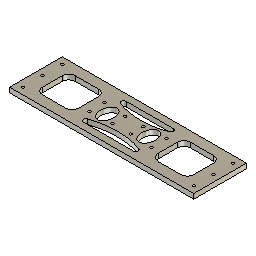
Mark3_new_z_vertical_bracket (Autodesk Fusion 360 design; units mm, degrees)
Autodesk Fusion 360 part; units mm, degrees
note: some values were not read from the file. Set by a fixed rule: which face or edge a step refers to.
sketch "Sketch1" plane through (0, 0, 0) normal (0, 0, 1) x (1, 0, 0)
  line L0 (17.5, -12.12) -> (-17.5, -12.12)
  line L1 (-17.5, -12.12) -> (-17.5, 12.12)
  line L2 (-17.5, 12.12) -> (17.5, 12.12)
  line L3 (17.5, 12.12) -> (17.5, -12.12)
  line L4 (17.5, -12.12) -> (-17.5, 12.12) construction
  line L5 (-17.5, -12.12) -> (17.5, 12.12) construction
  line L6 (114.3, -31.75) -> (-114.3, -31.75)
  line L7 (-114.3, -31.75) -> (-114.3, 31.75)
  line L8 (-114.3, 31.75) -> (114.3, 31.75)
  line L9 (114.3, 31.75) -> (114.3, -31.75)
  ellipse E0 centre (-38.75, 1.2425) end of major axis (-38.75, -20.9825) minor radius 13.97
  line L10 (-38.75, 23.4675) -> (-38.75, -20.9825)
  line L11 (-52.72, 1.2425) -> (-24.78, 1.2425)
  ellipse E1 centre (38.75, 1.2425) end of major axis (38.75, -20.9825) minor radius 13.97
  line L12 (38.75, 23.4675) -> (38.75, -20.9825)
  line L13 (24.78, 1.2425) -> (52.72, 1.2425)
  line L14 (635, -50.8) -> (279.4, -50.8)
  line L15 (279.4, -50.8) -> (279.4, 50.8)
  line L16 (279.4, 50.8) -> (635, 50.8)
  line L17 (635, 50.8) -> (635, -50.8)
  line L18 (635, -50.8) -> (279.4, 50.8) construction
  line L19 (279.4, -50.8) -> (635, 50.8) construction
  line L20 (381, -19.05) -> (381, 19.05)
  line L21 (533.4, 16.51) -> (533.4, -19.05)
  line L22 (533.4, -31.75) -> (381, 31.75) construction
  line L23 (381, -31.75) -> (533.4, 31.75) construction
  line L24 (311.15, 19.05) -> (311.15, -19.05)
  line L25 (603.25, -19.05) -> (603.25, 19.05)
  line L26 (603.25, 31.75) -> (311.15, -31.75) construction
  line L27 (311.15, 31.75) -> (603.25, -31.75) construction
  line L28 (590.55, 31.75) -> (548.64, 31.75)
  line L29 (368.3, 31.75) -> (323.85, 31.75)
  line L30 (323.85, -31.75) -> (368.3, -31.75)
  line L31 (546.1, -31.75) -> (590.55, -31.75)
  arc A0 (548.64, 31.75) -> (533.4, 16.51) centre (548.64, 16.51) ccw
  arc A1 (603.25, 19.05) -> (590.55, 31.75) centre (590.55, 19.05) ccw
  arc A2 (590.55, -31.75) -> (603.25, -19.05) centre (590.55, -19.05) ccw
  arc A3 (533.4, -19.05) -> (546.1, -31.75) centre (546.1, -19.05) ccw
  arc A4 (381, 19.05) -> (368.3, 31.75) centre (368.3, 19.05) ccw
  arc A5 (323.85, 31.75) -> (311.15, 19.05) centre (323.85, 19.05) ccw
  arc A6 (311.15, -19.05) -> (323.85, -31.75) centre (323.85, -19.05) ccw
  arc A7 (368.3, -31.75) -> (381, -19.05) centre (368.3, -19.05) ccw
  line L32 (457.2, -38.1) -> (528.32, -38.1)
  line L33 (457.2, -38.1) -> (393.7, -38.1)
  arc A8 (528.32, -38.1) -> (393.7, -38.1) centre (461.01, -156.5222) ccw
  line L34 (457.2, 38.1) -> (528.32, 38.1)
  line L35 (457.2, 38.1) -> (386.08, 38.1)
  arc A9 (386.08, 38.1) -> (528.32, 38.1) centre (457.2, 171.45) ccw
  ellipse E2 centre (418.45, 1.2425) end of major axis (418.45, -17.8075) minor radius 12.7
  line L36 (418.45, 20.2925) -> (418.45, -17.8075)
  line L37 (405.75, 1.2425) -> (431.15, 1.2425)
  ellipse E3 centre (495.95, -1.2425) end of major axis (495.95, -20.2925) minor radius 12.7
  line L38 (495.95, 17.8075) -> (495.95, -20.2925)
  line L39 (483.25, -1.2425) -> (508.65, -1.2425)
  point P0 (-60, 14.605)
  point P1 (-60, -14.605)
  point P2 (17.5, -12.12)
  point P3 (17.5, 12.12)
  point P4 (-17.5, 12.12)
  point P5 (-17.5, -12.12)
  point P6 (60, 14.605)
  point P7 (60, -14.605)
  point P8 (-114.3, 31.75)
  point P9 (114.3, 31.75)
  point P10 (114.3, -31.75)
  point P11 (-114.3, -31.75)
  point P12 (-38.75, 1.2425)
  point P13 (38.75, 1.2425)
  point P14 (457.2, 0)
  point P15 (517.2, 14.605)
  point P16 (517.2, -14.605)
  point P17 (439.7, -12.12)
  point P18 (397.2, -14.605)
  point P19 (397.2, 14.605)
  point P20 (474.7, -12.12)
  point P21 (474.7, 12.12)
  point P22 (457.2, 0)
  point P23 (457.2, 0)
  point P24 (439.7, 12.12)
  point P25 (457.2, 0)
  point P26 (418.45, 1.2425)
  point P27 (457.2, 0)
  point P28 (292.1, 38.1)
  point P29 (292.1, -38.1)
  point P30 (622.3, -38.1)
  point P31 (622.3, 38.1)
  point P32 (292.1, 0)
  point P33 (622.3, 0)
  point P34 (397.2, 14.605)
  point P35 (397.2, -14.605)
  point P36 (517.2, -14.605)
  point P37 (517.2, 14.605)
  point P38 (457.2, 0)
  point P39 (457.2, 0)
  point P40 (457.2, 0)
  point P41 (418.45, 1.2425)
  point P42 (495.95, -1.2425)
  point P43 (457.2, -50.8)
  point P44 (457.2, 50.8)
  dimension "d1" = 24.24
  dimension "d2" = 35
  dimension "d3" = 120
  dimension "d4" = 29.21
  dimension "d5" = 228.6
  dimension "d6" = 63.5
  dimension "d25" = 44.45
  dimension "d26" = 27.94
  dimension "d27" = 44.45
  dimension "d28" = 27.94
  dimension "d56" = 24.24
  dimension "d57" = 35
  dimension "d58" = 120
  dimension "d59" = 29.21
  dimension "d64" = 330.2
  dimension "d65" = 76.2
  dimension "d66" = 355.6
  dimension "d67" = 101.6
  dimension "d68" = 63.5
  dimension "d69" = 292.1
  dimension "d70" = 63.5
  dimension "d71" = 15.24
  dimension "d72" = 12.7
  dimension "d73" = 63.5
  dimension "d75" = 12.7
  dimension "d76" = 71.12
  dimension "d77" = 71.12
  dimension "d79" = 38.1
  dimension "d80" = 25.4
  dimension "d81" = 38.1
  dimension "d82" = 25.4
  constraint perpendicular L0 L1
  constraint parallel L0 L2
  constraint parallel L1 L3
  constraint horizontal L0
  constraint coincident L4 origin
  constraint coincident L5 origin
  constraint coincident P2 L0.start
  constraint coincident P3 L2.end
  constraint coincident P4 L1.end
  constraint coincident P5 L0.end
  constraint perpendicular L6 L7
  constraint parallel L6 L8
  constraint parallel L7 L9
  constraint horizontal L6
  constraint coincident P8 L7.end
  constraint coincident P9 L8.end
  constraint coincident P10 L6.start
  constraint coincident P11 L6.end
  constraint coincident P12 E0.centre
  constraint vertical L10
  constraint coincident E0 L10.start
  constraint coincident E0 L10.end
  constraint coincident E0 L11.start
  constraint coincident E0 L11.end
  constraint coincident P13 E1.centre
  constraint perpendicular L6 L12
  constraint coincident E1 L12.start
  constraint coincident E1 L12.end
  constraint coincident E1 L13.start
  constraint coincident E1 L13.end
  constraint coincident P40 P39
  constraint coincident P34 P19
  constraint coincident P35 P18
  constraint coincident P36 P16
  constraint coincident P15 P37
  constraint perpendicular L14 L15
  constraint parallel L14 L16
  constraint parallel L15 L17
  constraint horizontal L14
  constraint coincident L18 P40
  constraint coincident L19 P40
  constraint parallel L20 L21
  constraint coincident L22 P40
  constraint coincident L23 P40
  constraint perpendicular L24 L28
  constraint parallel L28 L30
  constraint parallel L24 L25
  constraint horizontal L28
  constraint coincident L26 P40
  constraint coincident L27 P40
  constraint collinear L28 L29
  constraint collinear L30 L31
  constraint coincident P41 P26
  constraint coincident L23.end L21
  constraint tangent L21 A0
  constraint tangent L28 A0
  constraint coincident L26.start L28
  constraint coincident L26.start L25
  constraint tangent L28 A1
  constraint tangent L25 A1
  constraint coincident L27.end L31
  constraint coincident L27.end L25
  constraint tangent L31 A2
  constraint tangent L25 A2
  constraint equal A1 A2
  constraint coincident L22.start L31
  constraint coincident L22.start L21
  constraint tangent L31 A3
  constraint tangent L21 A3
  constraint equal A1 A3
  constraint coincident L22.end L20
  constraint tangent L20 A4
  constraint tangent L29 A4
  constraint equal A1 A4
  constraint coincident L27.start L24
  constraint coincident L27.start L29
  constraint tangent L24 A5
  constraint tangent L29 A5
  constraint equal A1 A5
  constraint coincident L26.end L30
  constraint coincident L26.end L24
  constraint tangent L30 A6
  constraint tangent L24 A6
  constraint equal A1 A6
  constraint coincident L23.start L30
  constraint coincident L23.start L20
  constraint tangent L30 A7
  constraint tangent L20 A7
  constraint equal A1 A7
  constraint midpoint L14 P43
  constraint midpoint L16 P44
  constraint vertical L36
  constraint coincident E2 L36.start
  constraint coincident E2 L36.end
  constraint coincident E2 L37.start
  constraint coincident E2 L37.end
  constraint coincident P42 E3.centre
  constraint vertical L38
  constraint coincident E3 L38.start
  constraint coincident E3 L38.end
  constraint coincident E3 L39.start
  constraint coincident E3 L39.end
  measures "d1" distance of P5 P4
  measures "d2" distance of L1.end L2.end
  measures "d3" distance of P0 P6
  measures "d4" distance of P0 P1
  measures "d5" distance of P8 P9
  measures "d6" distance of P11 P8
  measures "d25" distance of E0
  measures "d27" distance of E1
  measures "d56" distance of P17 P24
  measures "d57" distance of P21 P24
  measures "d58" distance of P15 P34
  measures "d59" distance of P35 P34
  measures "d64" distance of P28 P31
  measures "d65" distance of P28 P29
  measures "d66" distance of L15.end L16.end
  measures "d67" distance of L14.end L15.end
  measures "d68" distance of L23.start L22.end
  measures "d69" distance of L26.end L27.end
  measures "d70" distance of L27.start L26.end
  measures "d71" radius of A0
  measures "d72" radius of A1
  measures "d73" distance of L32.start L33.end
  measures "d75" distance of P44 L34.start
  measures "d76" distance of L34.start L34.end
  measures "d77" distance of L34.start L35.end
  measures "d79" distance of E2
  measures "d81" distance of E3
extrude "Extrude1" add sketch "Sketch1" along normal blind 6.35 contours L0 L1 L2 L3 | L6 L7 L8 L9 | E0 L10 L11 | E0 L10 L11 | E0 L10 L11 | E0 L10 L11 | E1 L12 L13 | E1 L12 L13 | E1 L12 L13 | E1 L12 L13 makes body 1
hole "Hole1" at (60, 14.605, 0) at (-60, 14.605, 0) at (60, -14.605, 0) at (-60, -14.605, 0) at (-17.5, -12.12, 0) at (17.5, -12.12, 0) at (17.5, 12.12, 0) at (-17.5, 12.12, 0) direction (0, 0, 1) diameter 5 depth 75 tip angle 118 bodies 1
sketch "Sketch2" plane through (0, 0, 0) normal (0, 0, -1) x (1, 0, 0)
  circle A0 centre (17.5, -12.12) radius 2.5
  circle A1 centre (-17.5, 12.12) radius 2.5
  circle A2 centre (60, 14.605) radius 2.5
  circle A3 centre (60, -14.605) radius 2.5
  circle A4 centre (-60, -14.605) radius 2.5
  circle A5 centre (-60, 14.605) radius 2.5
  circle A6 centre (17.5, 12.12) radius 2.5
  circle A7 centre (-17.5, -12.12) radius 2.5
  line L0 (-114.3, -31.75) -> (114.3, -31.75)
  line L1 (114.3, -31.75) -> (114.3, 31.75)
  line L2 (114.3, 31.75) -> (-114.3, 31.75)
  line L3 (-114.3, 31.75) -> (-114.3, -31.75)
  line L4 (-88.2588, 0.0013) -> (-88.2621, -14.0439)
  line L5 (-88.2588, 0.0013) -> (-88.2577, 14.0481)
  line L6 (-82.1259, -19.0141) -> (-72.4219, -16.9514)
  line L7 (-82.1211, 19.0166) -> (-72.411, 16.9518)
  line L8 (-88.2572, 20.3213) -> (-67.964, 20.3213) construction
  line L9 (-68.3875, -16.0939) -> (-68.3875, 11.9829)
  line L10 (88.2885, 14.0454) -> (88.2779, -14.0541)
  line L11 (-88.2725, -20.3169) -> (-88.2572, 20.3213)
  line L12 (68.4111, 11.9838) -> (68.4022, -11.9841)
  line L13 (-68.3981, -11.9843) -> (-68.3875, 16.0963)
  line L14 (72.4255, -16.9549) -> (82.1413, -19.021)
  line L15 (72.435, 16.9509) -> (82.1524, 19.0163)
  arc A8 (-72.4219, -16.9514) -> (-68.3981, -11.9843) centre (-73.4781, -11.9824) ccw
  arc A9 (-68.3875, 11.9829) -> (-72.411, 16.9518) centre (-73.4675, 11.9829) ccw
  arc A10 (-82.1211, 19.0166) -> (-88.2577, 14.0481) centre (-83.1777, 14.0477) ccw
  arc A11 (-88.2621, -14.0439) -> (-82.1259, -19.0141) centre (-83.1821, -14.0451) ccw
  arc A12 (72.435, 16.9509) -> (68.4111, 11.9838) centre (73.4911, 11.9819) ccw
  arc A13 (68.4022, -11.9841) -> (72.4255, -16.9549) centre (73.4822, -11.986) ccw
  arc A14 (82.1413, -19.021) -> (88.2779, -14.0541) centre (83.1979, -14.0522) ccw
  arc A15 (88.2885, 14.0454) -> (82.1524, 19.0163) centre (83.2085, 14.0474) ccw
  point P0 (-97.7821, 20.7891)
  point P1 (97.809, 20.7899)
  point P2 (97.809, -20.7899)
  point P3 (-97.7855, -20.7849)
  point P4 (-97.7838, 0.0021)
  point P5 (97.809, 0)
  point P6 (-88.2635, -20.3187)
  point P7 (68.4006, -16.099)
  point P8 (88.2756, -20.3256)
  point P9 (68.4127, 16.0959)
  point P10 (88.2909, 20.3211)
  dimension "d15" = 9.525
  dimension "d16" = 20.32
  dimension "d17" = 20.32
  dimension "d19" = 20.32
  dimension "d22" = 5.08
  constraint horizontal L8
  constraint vertical L9
  constraint parallel L10 L11
  constraint parallel L12 L13
  constraint coincident L9.start L6
  constraint tangent L13 A8
  constraint tangent L6 A8
  constraint coincident L13.end L7
  constraint coincident L13.end L9
  constraint tangent L7 A9
  constraint tangent L9 A9
  constraint equal A8 A9
  constraint coincident L8.start L7
  constraint coincident L8.start L5
  constraint tangent L7 A10
  constraint tangent L5 A10
  constraint equal A8 A10
  constraint coincident P6 L4
  constraint coincident P6 L6
  constraint tangent L4 A11
  constraint tangent L6 A11
  constraint equal A8 A11
  constraint tangent L15 A12
  constraint tangent L12 A12
  constraint equal A8 A12
  constraint tangent L12 A13
  constraint tangent L14 A13
  constraint equal A8 A13
  constraint tangent L10 A14
  constraint tangent L14 A14
  constraint equal A8 A14
  constraint tangent L15 A15
  constraint tangent L10 A15
  constraint equal A8 A15
  measures "d15" distance of P4 L4.start
  measures "d16" distance of L4.start P6
  measures "d17" distance of L4.start L8.start
  measures "d19" distance of P6 L9.start
  measures "d22" radius of A8
extrude "Extrude2" cut sketch "Sketch2" against normal blind 15.24 contours L4 L5 L6 L7 L13 A8 A9 A10 A11 | L10 L12 L14 L15 A12 A13 A14 A15 bodies 1
extrude "Extrude3" cut sketch "Sketch1" along normal blind 12.7 contours E0 L10 L11 | E0 L10 L11 | E0 L10 L11 | E0 L10 L11 | E1 L12 L13 | E1 L12 L13 | E1 L12 L13 | E1 L12 L13 bodies 1
move_face "OffsetFaces1" offset 76.2 2 faces at (114.3, 10.5833, 2.1167) (-114.3, -10.5833, 2.1167) on bodies 1
sketch "Sketch3" plane through (0, 0, 6.35) normal (0, 0, 1) x (-1, 0, 0)
  ellipse E0 centre (-38.75, -1.2425) end of major axis (-38.75, 20.9825) minor radius 13.97
  ellipse E1 centre (38.75, -1.2425) end of major axis (38.75, 20.9825) minor radius 13.97
  arc A0 (82.1259, -19.0141) -> (88.2621, -14.0439) centre (83.1821, -14.0451) ccw
  line L0 (82.1259, -19.0141) -> (72.4219, -16.9514)
  arc A1 (68.3981, -11.9843) -> (72.4219, -16.9514) centre (73.4781, -11.9824) ccw
  line L1 (68.3981, -11.9843) -> (68.389, 12.1061)
  arc A2 (72.411, 16.9518) -> (68.389, 12.1061) centre (73.4675, 11.9829) ccw
  line L2 (72.411, 16.9518) -> (82.1211, 19.0166)
  arc A3 (88.2577, 14.0481) -> (82.1211, 19.0166) centre (83.1777, 14.0477) ccw
  line L3 (88.2577, 14.0481) -> (88.2588, 0.0013)
  line L4 (88.2588, 0.0013) -> (88.2621, -14.0439)
  line L5 (-68.4111, 11.9838) -> (-68.4022, -11.9841)
  arc A4 (-72.4255, -16.9549) -> (-68.4022, -11.9841) centre (-73.4822, -11.986) ccw
  line L6 (-72.4255, -16.9549) -> (-82.1413, -19.021)
  arc A5 (-88.2779, -14.0541) -> (-82.1413, -19.021) centre (-83.1979, -14.0522) ccw
  line L7 (-88.2779, -14.0541) -> (-88.2885, 14.0454)
  arc A6 (-82.1524, 19.0163) -> (-88.2885, 14.0454) centre (-83.2085, 14.0474) ccw
  line L8 (-82.1524, 19.0163) -> (-72.435, 16.9509)
  arc A7 (-68.4111, 11.9838) -> (-72.435, 16.9509) centre (-73.4911, 11.9819) ccw
  circle A8 centre (-17.5, -12.12) radius 2.5
  circle A9 centre (17.5, 12.12) radius 2.5
  circle A10 centre (-60, 14.605) radius 2.5
  circle A11 centre (-60, -14.605) radius 2.5
  circle A12 centre (60, -14.605) radius 2.5
  circle A13 centre (60, 14.605) radius 2.5
  circle A14 centre (-17.5, 12.12) radius 2.5
  circle A15 centre (17.5, -12.12) radius 2.5
  line L9 (-190.5, -31.75) -> (190.5, -31.75)
  line L10 (190.5, -31.75) -> (190.5, 31.75)
  line L11 (190.5, 31.75) -> (-190.5, 31.75)
  line L12 (-190.5, 31.75) -> (-190.5, -31.75)
  line L13 (-190.5, 0) -> (-180.975, 0)
  line L14 (-185.7375, 0) -> (-185.7375, -22.86)
  line L15 (-185.7375, 0) -> (-185.7375, 22.86)
  line L16 (190.5, 0) -> (180.975, 0)
  line L17 (185.7375, 0) -> (185.7375, -22.86)
  line L18 (185.7375, 0) -> (185.7375, 22.86)
  line L19 (88.2588, 0.0013) -> (113.6588, 0.0034)
  dimension "d32" = 9.525
  dimension "d33" = 22.86
  dimension "d34" = 22.86
  dimension "d35" = 9.525
  dimension "d36" = 22.86
  dimension "d37" = 22.86
  constraint midpoint L12 L13.start
  constraint perpendicular L12 L13
  constraint midpoint L13 L14.start
  constraint perpendicular L13 L14
  constraint perpendicular L13 L15
  constraint midpoint L10 L16.start
  constraint perpendicular L10 L16
  constraint midpoint L16 L17.start
  constraint perpendicular L16 L17
  constraint perpendicular L16 L18
  constraint coincident L3.end L4.start
  constraint perpendicular L3 L19
  measures "d32" distance of L13.start L13.end
  measures "d33" distance of L14.start L14.end
  measures "d34" distance of L14.start L15.end
  measures "d35" distance of L16.start L16.end
  measures "d36" distance of L17.start L17.end
  measures "d37" distance of L17.start L18.end
hole "Hole5" at (113.6832, 0.0139, 6.35) direction (0, 0, -1) diameter 38.1 depth 13.97 tip angle 118 bodies 1
hole "Hole3" at (-185.7375, 22.86, 6.35) direction (0, 0, -1) diameter 4.7498 depth 508 tip angle 118 bodies 1
hole "Hole4" at (-185.7375, -22.86, 6.35) at (185.7375, 22.86, 6.35) at (185.7375, -22.86, 6.35) at (-185.7375, 0, 6.35) at (185.7375, 0, 6.35) direction (0, 0, -1) diameter 4.7498 depth 13.97 tip angle 118 bodies 1
hole "Hole6" at (-113.6588, -0.0034, 6.35) direction (0, 0, -1) diameter 38.1 depth 13.97 tip angle 118 bodies 1
sketch "Sketch4" plane through (0, 0, 6.35) normal (0, 0, 1) x (-1, 0, 0)
  circle A0 centre (113.6588, 0.0034) radius 19.05
  circle A1 centre (185.7375, 0) radius 2.3749
  circle A2 centre (-185.7375, -22.86) radius 2.3749
  circle A3 centre (185.7375, 22.86) radius 2.3749
  circle A4 centre (-185.7375, 22.86) radius 2.3749
  circle A5 centre (-185.7375, 0) radius 2.3749
  circle A6 centre (185.7375, -22.86) radius 2.3749
  circle A7 centre (-113.6832, -0.0139) radius 19.05
  ellipse E0 centre (-38.75, -1.2425) end of major axis (-38.75, 20.9825) minor radius 13.97
  ellipse E1 centre (38.75, -1.2425) end of major axis (38.75, 20.9825) minor radius 13.97
  arc A8 (82.1259, -19.0141) -> (88.2621, -14.0439) centre (83.1821, -14.0451) ccw
  line L0 (82.1259, -19.0141) -> (72.4219, -16.9514)
  arc A9 (68.3981, -11.9843) -> (72.4219, -16.9514) centre (73.4781, -11.9824) ccw
  line L1 (68.3981, -11.9843) -> (68.389, 12.1061)
  arc A10 (72.411, 16.9518) -> (68.389, 12.1061) centre (73.4675, 11.9829) ccw
  line L2 (72.411, 16.9518) -> (82.1211, 19.0166)
  arc A11 (88.2577, 14.0481) -> (82.1211, 19.0166) centre (83.1777, 14.0477) ccw
  line L3 (88.2577, 14.0481) -> (88.2588, 0.0013)
  line L4 (88.2588, 0.0013) -> (88.2621, -14.0439)
  line L5 (-68.4111, 11.9838) -> (-68.4022, -11.9841)
  arc A12 (-72.4255, -16.9549) -> (-68.4022, -11.9841) centre (-73.4822, -11.986) ccw
  line L6 (-72.4255, -16.9549) -> (-82.1413, -19.021)
  arc A13 (-88.2779, -14.0541) -> (-82.1413, -19.021) centre (-83.1979, -14.0522) ccw
  line L7 (-88.2779, -14.0541) -> (-88.2885, 14.0454)
  arc A14 (-82.1524, 19.0163) -> (-88.2885, 14.0454) centre (-83.2085, 14.0474) ccw
  line L8 (-82.1524, 19.0163) -> (-72.435, 16.9509)
  arc A15 (-68.4111, 11.9838) -> (-72.435, 16.9509) centre (-73.4911, 11.9819) ccw
  circle A16 centre (-17.5, -12.12) radius 2.5
  circle A17 centre (17.5, 12.12) radius 2.5
  circle A18 centre (-60, 14.605) radius 2.5
  circle A19 centre (-60, -14.605) radius 2.5
  circle A20 centre (60, -14.605) radius 2.5
  circle A21 centre (60, 14.605) radius 2.5
  circle A22 centre (-17.5, 12.12) radius 2.5
  circle A23 centre (17.5, -12.12) radius 2.5
  line L9 (-190.5, -31.75) -> (190.5, -31.75)
  line L10 (190.5, -31.75) -> (190.5, 31.75)
  line L11 (190.5, 31.75) -> (-190.5, 31.75)
  line L12 (-190.5, 31.75) -> (-190.5, -31.75)
  circle A24 centre (-156.5366, 0) radius 15.875
  circle A25 centre (156.8419, 0) radius 15.875
  point P0 (180.975, 0)
  dimension "d52" = 31.75
  dimension "d53" = 31.75
  measures "d52" diameter of A24
  measures "d53" diameter of A25
extrude "Extrude4" cut sketch "Sketch4" against normal blind 38.1 contours A24 | A25 bodies 1
extrude "Extrude5" add sketch "Sketch1" along normal blind 9.525 separate body contours L14 L15 L16 L17 makes body 2
fillet "Fillet1" radius 4.826 1 edges at (386.08, 38.1, 4.7625) on bodies 2
fillet "Fillet2" radius 4.826 3 edges at (528.32, 38.1, 4.7625) (528.32, -38.1, 4.7625) (393.7, -38.1, 4.7625) on bodies 2
sketch "Sketch5" plane through (0, 0, 9.525) normal (0, 0, 1) x (-1, 0, 0)
  arc A0 (-533.4, 19.05) -> (-546.1, 31.75) centre (-546.1, 19.05) ccw
  line L0 (-533.4, 19.05) -> (-533.4, -16.51)
  arc A1 (-548.64, -31.75) -> (-533.4, -16.51) centre (-548.64, -16.51) ccw
  line L1 (-548.64, -31.75) -> (-590.55, -31.75)
  arc A2 (-603.25, -19.05) -> (-590.55, -31.75) centre (-590.55, -19.05) ccw
  line L2 (-603.25, -19.05) -> (-603.25, 19.05)
  arc A3 (-590.55, 31.75) -> (-603.25, 19.05) centre (-590.55, 19.05) ccw
  line L3 (-590.55, 31.75) -> (-546.1, 31.75)
  arc A4 (-368.3, 31.75) -> (-381, 19.05) centre (-368.3, 19.05) ccw
  line L4 (-368.3, 31.75) -> (-323.85, 31.75)
  arc A5 (-311.15, 19.05) -> (-323.85, 31.75) centre (-323.85, 19.05) ccw
  line L5 (-311.15, 19.05) -> (-311.15, -19.05)
  arc A6 (-323.85, -31.75) -> (-311.15, -19.05) centre (-323.85, -19.05) ccw
  line L6 (-323.85, -31.75) -> (-368.3, -31.75)
  arc A7 (-381, -19.05) -> (-368.3, -31.75) centre (-368.3, -19.05) ccw
  line L7 (-381, -19.05) -> (-381, 19.05)
  line L8 (-506.5389, 38.1) -> (-415.4811, 38.1)
  arc A8 (-413.8088, 28.747) -> (-415.4811, 38.1) centre (-415.4811, 33.274) ccw
  arc A9 (-508.2112, 28.747) -> (-413.8088, 28.747) centre (-461.01, 156.5222) ccw
  arc A10 (-506.5389, 38.1) -> (-508.2112, 28.747) centre (-506.5389, 33.274) ccw
  ellipse E0 centre (-418.45, -1.2425) end of major axis (-418.45, 17.8075) minor radius 12.7
  line L9 (-409.1141, -38.1) -> (-505.2859, -38.1)
  arc A11 (-506.8721, -28.7161) -> (-505.2859, -38.1) centre (-505.2859, -33.274) ccw
  arc A12 (-407.5279, -28.7161) -> (-506.8721, -28.7161) centre (-457.2, -171.45) ccw
  arc A13 (-409.1141, -38.1) -> (-407.5279, -28.7161) centre (-409.1141, -33.274) ccw
  ellipse E1 centre (-495.95, 1.2425) end of major axis (-495.95, 20.2925) minor radius 12.7
  line L10 (-635, -50.8) -> (-279.4, -50.8)
  line L11 (-279.4, -50.8) -> (-279.4, 50.8)
  line L12 (-279.4, 50.8) -> (-635, 50.8)
  line L13 (-635, 50.8) -> (-635, -50.8)
hole "Hole7" at (622.3, 38.1, 0) direction (0, 0, 1) diameter 5 depth 60 tip angle 118 bodies 2
hole "Hole8" at (622.3, 0, 0) at (622.3, -38.1, 0) at (517.2, -14.605, 0) at (517.2, 14.605, 0) at (474.7, 12.12, 0) at (474.7, -12.12, 0) at (439.7, -12.12, 0) at (439.7, 12.12, 0) at (397.2, 14.605, 0) at (397.2, -14.605, 0) at (292.1, -38.1, 0) at (292.1, 0, 0) at (292.1, 38.1, 0) direction (0, 0, 1) diameter 5 depth 60 tip angle 118 bodies 2
sketch "Sketch6" plane through (0, 0, 0) normal (0, 0, -1) x (1, 0, 0)
  circle A0 centre (292.1, 0) radius 2.5
  circle A1 centre (397.2, 14.605) radius 2.5
  circle A2 centre (439.7, -12.12) radius 2.5
  circle A3 centre (474.7, 12.12) radius 2.5
  circle A4 centre (517.2, -14.605) radius 2.5
  circle A5 centre (622.3, 38.1) radius 2.5
  circle A6 centre (622.3, 0) radius 2.5
  circle A7 centre (517.2, 14.605) radius 2.5
  circle A8 centre (474.7, -12.12) radius 2.5
  circle A9 centre (439.7, 12.12) radius 2.5
  circle A10 centre (397.2, -14.605) radius 2.5
  circle A11 centre (292.1, 38.1) radius 2.5
  circle A12 centre (292.1, -38.1) radius 2.5
  circle A13 centre (622.3, -38.1) radius 2.5
  arc A14 (546.1, 31.75) -> (533.4, 19.05) centre (546.1, 19.05) ccw
  line L0 (546.1, 31.75) -> (590.55, 31.75)
  arc A15 (603.25, 19.05) -> (590.55, 31.75) centre (590.55, 19.05) ccw
  line L1 (603.25, 19.05) -> (603.25, -19.05)
  arc A16 (590.55, -31.75) -> (603.25, -19.05) centre (590.55, -19.05) ccw
  line L2 (590.55, -31.75) -> (548.64, -31.75)
  arc A17 (533.4, -16.51) -> (548.64, -31.75) centre (548.64, -16.51) ccw
  line L3 (533.4, -16.51) -> (533.4, 19.05)
  arc A18 (381, 19.05) -> (368.3, 31.75) centre (368.3, 19.05) ccw
  line L4 (381, 19.05) -> (381, -19.05)
  arc A19 (368.3, -31.75) -> (381, -19.05) centre (368.3, -19.05) ccw
  line L5 (368.3, -31.75) -> (323.85, -31.75)
  arc A20 (311.15, -19.05) -> (323.85, -31.75) centre (323.85, -19.05) ccw
  line L6 (311.15, -19.05) -> (311.15, 19.05)
  arc A21 (323.85, 31.75) -> (311.15, 19.05) centre (323.85, 19.05) ccw
  line L7 (323.85, 31.75) -> (368.3, 31.75)
  arc A22 (508.2112, 28.747) -> (506.5389, 38.1) centre (506.5389, 33.274) ccw
  arc A23 (413.8088, 28.747) -> (508.2112, 28.747) centre (461.01, 156.5222) ccw
  arc A24 (415.4811, 38.1) -> (413.8088, 28.747) centre (415.4811, 33.274) ccw
  line L8 (415.4811, 38.1) -> (506.5389, 38.1)
  ellipse E0 centre (418.45, -1.2425) end of major axis (418.45, 17.8075) minor radius 12.7
  arc A25 (407.5279, -28.7161) -> (409.1141, -38.1) centre (409.1141, -33.274) ccw
  arc A26 (506.8721, -28.7161) -> (407.5279, -28.7161) centre (457.2, -171.45) ccw
  arc A27 (505.2859, -38.1) -> (506.8721, -28.7161) centre (505.2859, -33.274) ccw
  line L9 (505.2859, -38.1) -> (409.1141, -38.1)
  ellipse E1 centre (495.95, 1.2425) end of major axis (495.95, 20.2925) minor radius 12.7
  line L10 (279.4, -50.8) -> (635, -50.8)
  line L11 (635, -50.8) -> (635, 50.8)
  line L12 (635, 50.8) -> (279.4, 50.8)
  line L13 (279.4, 50.8) -> (279.4, -50.8)
  line L14 (690.5625, -50.8) -> (681.0375, -50.8)
  line L15 (681.0375, -50.8) -> (681.0375, 50.8)
  line L16 (681.0375, 50.8) -> (690.5625, 50.8)
  line L17 (690.5625, 50.8) -> (690.5625, -50.8)
  line L18 (690.5625, -50.8) -> (681.0375, 50.8) construction
  line L19 (681.0375, -50.8) -> (690.5625, 50.8) construction
  point P0 (685.8, 0)
  dimension "d93" = 101.6
  dimension "d94" = 9.525
  constraint perpendicular L14 L15
  constraint parallel L14 L16
  constraint parallel L15 L17
  constraint horizontal L14
  constraint coincident L18 P0
  constraint coincident L19 P0
  measures "d93" distance of L14.end L15.end
  measures "d94" distance of L15.end L16.end
sketch "Sketch14" plane through (690.5625, 0, 0) normal (1, 0, 0) x (0, 1, 0)
  line L0 (50.8, 0) -> (-50.8, 0)
  line L1 (-50.8, 0) -> (-50.8, -304.8)
  line L2 (-50.8, -304.8) -> (50.8, -304.8)
  line L3 (50.8, -304.8) -> (50.8, 0)
  line L4 (-50.8, 0) -> (50.8, 0)
  line L5 (-50.8, 0) -> (-50.8, -304.8)
  line L6 (50.8, 0) -> (50.8, 7.4245)
  line L7 (-50.8, -304.8) -> (0, -304.8)
  ellipse E0 centre (-7.62, -81.28) end of major axis (-3.4023, -30.6672) minor radius 28.8705
  ellipse E1 centre (-15.24, -182.88) end of major axis (-18.4769, -221.7224) minor radius 17.7909
  ellipse E2 centre (-22.86, -259.08) end of major axis (-24.9978, -284.7341) minor radius 12.0882
  line L8 (-50.8, -304.8) -> (0, -304.8)
  line L9 (0, -304.8) -> (0, -295.275)
  line L10 (-50.8, -295.275) -> (-50.8, -304.8)
  line L11 (50.8, 0) -> (50.8, -25.4)
  arc A0 (50.8, -25.4) -> (0, -295.275) centre (3171.3517, -752.5166) ccw
  point P0 (0, -295.275)
  dimension "d129" = 50.8
  dimension "d134" = 25.4
  constraint coincident L0.end L1.start
  constraint coincident L0.start L3.end
  constraint coincident L1.end L2.start
  constraint perpendicular L1 L7
  constraint perpendicular L8 L9
  constraint parallel L9 L10
  constraint horizontal L8
  constraint coincident P0 L9.end
  constraint perpendicular L4 L11
  measures "d129" distance of L1.end L7.end
  measures "d134" distance of L0.start L11.end
extrude "Extrude14" add sketch "Sketch14" against normal blind 9.525 separate body contours L0 L1 L2 L3 L4 L5 L7 L8 L9 L10 L11 A0 makes body 3
copy_body "CopyPasteBodies3" bodies 3 makes body 4
move_body "Move4" bodies 4 to x (1, 0, 0) y (0, 1, 0) z (0, 0, 1) at (-406.4, 0, 0)
move_body "Move5" bodies 3 to x (1, 0, 0) y (0, 1, 0) z (0, 0, 1) at (-57.15, 0, 0)
move_body "Move6" bodies 2 to x (1, 0, 0) y (0, 1, 0) z (0, 0, 1) at (0, 0, 38.1)
move_body "Align1" bodies 2 to x (1, 0, 0) y (0, 1, 0) z (0, 0, 1) at (-4.7625, 0, -38.1)
move_body "Move7" bodies 3 to x (1, 0, 0) y (0, 1, 0) z (0, 0, 1) at (0, 0, -25.4)
move_body "Align2" bodies 3 to x (1, 0, 0) y (0, 1, 0) z (0, 0, 1) at (-3.175, 0, 25.4)
sketch "Sketch15" plane through (630.2375, 0, 0) normal (1, 0, 0) x (0, 1, 0)
  ellipse E0 centre (-15.24, -182.88) end of major axis (-18.4769, -221.7224) minor radius 17.7909
  ellipse E1 centre (-22.86, -259.08) end of major axis (-24.9978, -284.7341) minor radius 12.0882
  ellipse E2 centre (-7.62, -81.28) end of major axis (-3.4023, -30.6672) minor radius 28.8705
  line L0 (-50.8, 0) -> (-50.8, -304.8)
  line L1 (-50.8, -304.8) -> (0, -304.8)
  line L2 (0, -304.8) -> (0, -295.275)
  arc A0 (50.8, -25.4) -> (0, -295.275) centre (3171.3517, -752.5166) ccw
  line L3 (50.8, -25.4) -> (50.8, 0)
  line L4 (50.8, 0) -> (-50.8, 0)
  line L5 (-50.8, -304.8) -> (0, -304.8)
  line L6 (0, -304.8) -> (0, -295.275)
  line L7 (0, -295.275) -> (-50.8, -295.275)
  line L8 (-50.8, -295.275) -> (-50.8, -304.8)
  line L9 (-50.8, -300.0375) -> (-38.1, -300.0375)
  line L10 (0, -300.0375) -> (-12.7, -300.0375)
  line L11 (-12.7, -300.0375) -> (-38.1, -300.0375)
  point P0 (-25.4, -300.0375)
  point P1 (-38.1, -300.0375)
  point P2 (-12.7, -300.0375)
  dimension "d137" = 12.7
  dimension "d138" = 12.7
  constraint horizontal L5
  constraint vertical L6
  constraint horizontal L7
  constraint vertical L8
  constraint coincident L2.end A0.end
  constraint coincident L0.end L1.start
  constraint midpoint L8 L9.start
  constraint perpendicular L8 L9
  constraint midpoint L6 L10.start
  constraint perpendicular L6 L10
  constraint midpoint L11 P0
  constraint coincident P1 L9.end
  constraint coincident P2 L10.end
  measures "d137" distance of L9.start P1
  measures "d138" distance of L10.start P2
hole "Hole11" at (630.2375, -12.7, -300.0375) direction (-1, 0, 0) diameter 5 depth 500 tip angle 118 bodies 3 4
hole "Hole12" at (630.2375, -25.4, -300.0375) at (630.2375, -38.1, -300.0375) direction (-1, 0, 0) diameter 5 depth 500 tip angle 118 bodies 3 4
sketch "Sketch16" plane through (0, -50.8, 0) normal (0, -1, 0) x (1, 0, 0)
  line L0 (284.1625, -304.8) -> (284.1625, 0)
  line L1 (284.1625, 0) -> (274.6375, 0)
  line L2 (274.6375, 0) -> (274.6375, -304.8)
  line L3 (274.6375, -304.8) -> (284.1625, -304.8)
  line L4 (284.1625, -304.8) -> (620.7125, -304.8)
  line L5 (620.7125, -304.8) -> (620.7125, -314.325)
  line L6 (620.7125, -314.325) -> (284.1625, -314.325)
  line L7 (284.1625, -314.325) -> (284.1625, -304.8)
  dimension "d145" = 336.55
  dimension "d146" = 9.525
  constraint horizontal L4
  constraint vertical L5
  constraint horizontal L6
  constraint vertical L7
  constraint coincident L0.start L3.end
  measures "d145" distance of L0.start L4.end
  measures "d146" distance of L0.start L6.end
extrude "Extrude15" add sketch "Sketch16" against normal blind 50.8 separate body contours L4 L5 L6 L7 makes body 5
sketch "Sketch17" plane through (0, 0, -314.325) normal (0, 0, -1) x (1, 0, 0)
  line L0 (620.7125, 50.8) -> (284.1625, 50.8)
  line L1 (284.1625, 50.8) -> (284.1625, 0)
  line L2 (284.1625, 0) -> (620.7125, 0)
  line L3 (620.7125, 0) -> (620.7125, 50.8)
  ellipse E0 centre (536.575, 25.4) end of major axis (581.025, 25.4) minor radius 15.875
  line L4 (492.125, 25.4) -> (581.025, 25.4)
  line L5 (536.575, 9.525) -> (536.575, 41.275)
  ellipse E1 centre (368.3, 25.4) end of major axis (412.75, 25.4) minor radius 15.875
  line L6 (323.85, 25.4) -> (412.75, 25.4)
  line L7 (368.3, 9.525) -> (368.3, 41.275)
  ellipse E2 centre (304.0062, 25.4) end of major axis (304.0062, 9.525) minor radius 9.525
  line L8 (304.0062, 41.275) -> (304.0062, 9.525)
  ellipse E3 centre (600.8687, 25.4) end of major axis (600.8687, 9.525) minor radius 9.525
  line L9 (600.8687, 41.275) -> (600.8687, 9.525)
  ellipse E4 centre (452.4375, 25.4) end of major axis (471.4875, 25.4) minor radius 12.7
  line L10 (433.3875, 25.4) -> (471.4875, 25.4)
  line L11 (452.4375, 12.7) -> (452.4375, 38.1)
  point P0 (452.4375, 25.4)
  point P1 (368.3, 25.4)
  point P2 (536.575, 25.4)
  point P3 (304.0062, 25.4)
  point P4 (600.8687, 25.4)
  dimension "d149" = 88.9
  dimension "d150" = 31.75
  dimension "d151" = 88.9
  dimension "d152" = 31.75
  dimension "d153" = 31.75
  dimension "d154" = 19.05
  dimension "d155" = 31.75
  dimension "d156" = 19.05
  dimension "d159" = 38.1
  dimension "d160" = 25.4
  constraint coincident P2 E0.centre
  constraint coincident E0 L4.start
  constraint coincident E0 L4.end
  constraint coincident E0 L5.start
  constraint coincident E0 L5.end
  constraint coincident P1 E1.centre
  constraint coincident E1 L6.start
  constraint coincident E1 L6.end
  constraint coincident E1 L7.start
  constraint coincident E1 L7.end
  constraint coincident P3 E2.centre
  constraint coincident E2 L8.start
  constraint coincident E2 L8.end
  constraint coincident P4 E3.centre
  constraint coincident E3 L9.start
  constraint coincident E3 L9.end
  constraint coincident P0 E4.centre
  constraint horizontal L10
  constraint coincident E4 L10.start
  constraint coincident E4 L10.end
  constraint coincident E4 L11.start
  constraint coincident E4 L11.end
  measures "d149" distance of E0
  measures "d151" distance of E1
  measures "d153" distance of E2
  measures "d155" distance of E3
  measures "d159" distance of E4
extrude "Extrude17" cut sketch "Sketch17" against normal blind 12.7 contours E4 L10 L11 | E4 L10 L11 | E4 L10 L11 | E4 L10 L11 bodies 5
extrude "Extrude16" cut sketch "Sketch17" against normal blind 22.86 contours E0 L4 L5 | E0 L4 L5 | E0 L4 L5 | E0 L4 L5 | E1 L6 L7 | E1 L6 L7 | E1 L6 L7 | E1 L6 L7 | E2 L8 | E2 L8 | E3 L9 | E3 L9 bodies 5
move_body "Move8" bodies 5 to x (1, 0, 0) y (0, 1, 0) z (0, 0, 1) at (0, 0, -50.8)
move_body "Align3" bodies 5 to x (1, 0, 0) y (0, 1, 0) z (0, 0, 1) at (0, 0, 60.325)
sketch "Sketch18" plane through (0, -50.8, 0) normal (0, -1, 0) x (1, 0, 0)
  line L0 (284.1625, -304.8) -> (284.1625, 0)
  line L1 (284.1625, 0) -> (274.6375, 0)
  line L2 (274.6375, 0) -> (274.6375, -304.8)
  line L3 (274.6375, -304.8) -> (284.1625, -304.8)
  line L4 (630.2375, 0) -> (620.7125, 0)
  line L5 (284.1625, -152.4) -> (622.3, -152.4)
  point P0 (279.4, -40.4829)
  point P1 (279.4, -40.4829)
  point P2 (630.2375, 0)
  point P3 (625.475, -40.4829)
  point P4 (625.475, -40.4829)
  point P5 (453.2312, -152.4)
  constraint coincident P1 P0
  constraint coincident P2 L4.start
  constraint coincident P4 P3
  constraint midpoint L0 L5.start
  constraint perpendicular L0 L5
  constraint midpoint L5 P5
sketch "Sketch19" plane through (0, -50.8, 0) normal (0, -1, 0) x (1, 0, 0)
  line L0 (284.1625, -304.8) -> (620.7125, -304.8)
  line L1 (620.7125, -304.8) -> (620.7125, -295.275)
  line L2 (620.7125, -295.275) -> (284.1625, -295.275)
  line L3 (284.1625, -295.275) -> (284.1625, -304.8)
  circle A0 centre (452.4375, -300.0375) radius 2
  point P0 (452.4375, -300.0375)
  point P1 (452.4375, -300.0375)
  dimension "d169" = 4
  constraint coincident P1 P0
  measures "d169" diameter of A0
extrude "Extrude18" add sketch "Sketch19" along normal blind 5 separate body contours A0 makes body 6
hole "Hole14" at (452.4375, -50.8, -300.0375) direction (0, 1, 0) diameter 4 depth 20 tip angle 118 bodies 5
extrude "Extrude19" add sketch "Sketch19" against normal blind 12 contours A0 bodies 6
thread "Thread1" "ISO Metric profile 4.0 M4x0.7 6g" major diameter 3.908 minor diameter 3.111 pitch 0.7 angle 60 modelled right hand crest width 0.1017 on face at (454.3756, -54.1333, -299.544) crest through (454.3915, -38.625, -300.0375) on face at (454.3756, -42.8, -299.544) crest through (454.3915, -38.625, -300.0375) on bodies 6
sphere "SpherePrimitive1" add diameter 10 placed x (1, 0, 0) y (0, 0, 1) z (0, -1, 0) at (452.4375, -55.8, -300.0375) bodies 6
copy_body "CopyPasteBodies4" bodies 6 makes body 7
move_body "Move9" bodies 7 to x (1, 0, 0) y (0, 1, 0) z (0, 0, 1) at (0, 0, 59)
copy_body "CopyPasteBodies5" bodies 6 makes body 8
move_body "Move10" bodies 8 to x (1, 0, 0) y (0, 1, 0) z (0, 0, 1) at (0, 0, 40)
move_body "Align4" bodies 6 to x (1, 0, 0) y (0, 1, 0) z (0, 0, 1) at (173.0375, -12, 259.5546)
move_body "Align5" bodies 8 to x (1, 0, 0) y (0, 1, 0) z (0, 0, 1) at (-173.0382, -12, 219.4216)
move_body "Align6" bodies 7 to x (1, 0, 0) y (0, 1, 0) z (0, 0, 1) at (-0.0007, -12, -59.133)
move_body "Move11" bodies 8 7 6 to x (1, 0, 0) y (0, 1, 0) z (0, 0, 1) at (0, 10, 0)
sketch "Sketch21" plane through (0, -50.8, 0) normal (0, -1, 0) x (1, 0, 0)
  line L0 (274.6375, 0) -> (630.2375, 0)
  line L1 (630.2375, 0) -> (630.2375, 9.525)
  line L2 (630.2375, 9.525) -> (274.6375, 9.525)
  line L3 (274.6375, 9.525) -> (274.6375, 0)
  circle A0 centre (460, 50) radius 6
  dimension "d175" = 12
  measures "d175" diameter of A0
extrude "Extrude20" add sketch "Sketch21" along normal blind 10 separate body contours A0 makes body 9
sphere "SpherePrimitive2" cut diameter 10 placed x (1, 0, 0) y (0, 0, 1) z (0, -1, 0) at (460, -50.8, 50) bodies 9
hole "Hole15" at (460, -50.8, 50) direction (0, -1, 0) diameter 4 depth 20 tip angle 118 bodies 9
copy_body "CopyPasteBodies6" bodies 9 makes body 10
move_body "Move12" bodies 10 to x (1, 0, 0) y (0, 1, 0) z (0, 0, 1) at (85, 0, 0)
copy_body "CopyPasteBodies7" bodies 9 makes body 11
move_body "Move13" bodies 11 to x (1, 0, 0) y (0, 1, 0) z (0, 0, 1) at (40, 0, 0)
move_body "Align7" bodies 10 to x (1, 0, 0) y (0, 1, 0) z (0, 0, 1) at (-265.6, 0, -90.4829)
move_body "Move14" bodies 10 to x (1, 0, 0) y (0, 1, 0) z (0, 0, 1) at (0, -8, 0)
move_body "Align8" bodies 9 to x (1, 0, 0) y (0, 1, 0) z (0, 0, 1) at (165.475, 0, -90.4829)
move_body "Move15" bodies 9 to x (1, 0, 0) y (0, 1, 0) z (0, 0, 1) at (0, -8, 0)
move_body "Align9" bodies 11 to x (1, 0, 0) y (0, 1, 0) z (0, 0, 1) at (-47.5625, 0, -350.0375)
move_body "Move16" bodies 11 to x (1, 0, 0) y (0, 1, 0) z (0, 0, 1) at (0, -8, 0)
sketch "Sketch23" plane through (0, -50.8, 0) normal (0, -1, 0) x (1, 0, 0)
sketch "Sketch24" plane through (0, -50.8, 0) normal (0, -1, 0) x (1, 0, 0)
  line L0 (630.2375, -304.8) -> (630.2375, 0)
  line L1 (630.2375, 0) -> (620.7125, 0)
  line L2 (620.7125, 0) -> (620.7125, -304.8)
  line L3 (620.7125, -304.8) -> (630.2375, -304.8)
  line L4 (1130.3, -88.9) -> (723.9, -88.9)
  line L5 (723.9, -88.9) -> (723.9, 215.9)
  line L6 (723.9, 215.9) -> (1130.3, 215.9)
  line L7 (1130.3, 215.9) -> (1130.3, -88.9)
  line L8 (1130.3, -88.9) -> (723.9, 215.9) construction
  line L9 (723.9, -88.9) -> (1130.3, 215.9) construction
  point P0 (927.1, 63.5)
  dimension "d182" = 406.4
  dimension "d183" = 304.8
  constraint perpendicular L4 L5
  constraint parallel L4 L6
  constraint parallel L5 L7
  constraint horizontal L4
  constraint coincident L8 P0
  constraint coincident L9 P0
  measures "d182" distance of L5.end L6.end
  measures "d183" distance of L4.end L5.end
extrude "Extrude21" add sketch "Sketch24" along normal blind 6.35 separate body contours L4 L5 L6 L7 makes body 12
move_body "Align10" bodies 12 to x (1, 0, 0) y (0, 1, 0) z (0, 0, 1) at (-473.8687, 6.35, -215.9)
move_body "Move17" bodies 12 to x (1, 0, 0) y (0, 1, 0) z (0, 0, 1) at (0, -24.384, 0)
move_face "OffsetFaces4" offset 10.16 1 faces at (385.4979, -70.9507, 0) on bodies 12
move_face "OffsetFaces5" offset 2.54 1 faces at (520.9646, -70.9507, -304.8) on bodies 12
move_body "Move18" bodies 7 12 2 10 9 11 3 4 5 6 8 to x (1, 0, 0) y (0, 0, -1) z (0, 1, 0) at (0, 79.756, -217.424)
move_body "Move19" bodies 2 to x (1, 0, 0) y (0, 0, -1) z (0, 1, 0) at (0, 347.98, -188.468)
move_body "Align11" bodies 2 to x (1, 0, 0) y (0, 1, 0) z (0, 0, 1) at (-274.6375, -79.756, 268.224)
sketch "Sketch7" plane through (681.0375, 0, 0) normal (-1, 0, 0) x (0, -1, 0)
  line L0 (50.8, 0) -> (-50.8, 0)
  line L1 (-50.8, 0) -> (-50.8, -304.8)
  line L2 (-50.8, -304.8) -> (50.8, -304.8)
  line L3 (50.8, -304.8) -> (50.8, 0)
  line L4 (50.8, -304.8) -> (25.4, -304.8)
  line L5 (-50.8, 0) -> (-50.8, -50.8)
  line L6 (-50.8, -50.8) -> (-50.8, -304.8)
  line L7 (25.4, -304.8) -> (-50.8, -304.8)
  dimension "d97" = 25.4
  constraint coincident L2.end L3.start
  constraint perpendicular L3 L4
  constraint coincident L0.end L1.start
  constraint coincident L1 L5.end
  constraint coincident L1.end L2.start
  measures "d97" distance of L2.end L4.end
hidden bodies 1 3 4 5 6 7 8 9 10 11 12
